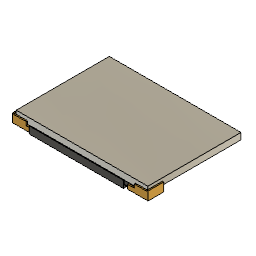
Brackets for Speaker Stand v2 (Autodesk Fusion 360 design; units mm, degrees)
part number: 2026-08-03-13-08-30-619
Autodesk Fusion 360 part; units mm, degrees
sketch "sk REF plate sheet" plane through (0, 0, 0) normal (0, 0, 1) x (1, 0, 0)
  line L0 (-111.75, -122.5) -> (111.75, -122.5)
  line L1 (111.75, -122.5) -> (111.75, 122.5)
  line L2 (111.75, 122.5) -> (-111.75, 122.5)
  line L3 (-111.75, 122.5) -> (-111.75, -122.5)
  dimension "d100" = 111.75
  dimension "d101" = 122.5
  dimension "d102" = 111.75
  dimension "d103" = 122.5
  measures "d100" horizontal distance of origin L0.start
  measures "d101" vertical distance of origin L0.start
  measures "d102" horizontal distance of origin L1.end
  measures "d103" vertical distance of origin L1.end
extrude "REF plate sheet" add sketch "sk REF plate sheet" along normal blind 1.8 makes body 1
sketch "sk REF plate lip" plane through (0, 0, 0) normal (0, 0, 1) x (1, 0, 0)
  line L0 (-111.75, -122.5) -> (111.75, -122.5)
  line L1 (111.75, -122.5) -> (111.75, -120.7)
  line L2 (111.75, -120.7) -> (-111.75, -120.7)
  line L3 (-111.75, -120.7) -> (-111.75, -122.5)
  dimension "d107" = 111.75
  dimension "d108" = 122.5
  dimension "d109" = 111.75
  dimension "d110" = 120.7
  measures "d107" horizontal distance of origin L0.start
  measures "d108" vertical distance of origin L0.start
  measures "d109" horizontal distance of origin L1.end
  measures "d110" vertical distance of origin L1.end
extrude "REF plate lip" add sketch "sk REF plate lip" along normal blind 16.8 bodies 1
fillet "REF plate rear corners" radius 14 2 edges at (111.75, 122.5, 0.9) (-111.75, 122.5, 0.9) on bodies 1
fillet "REF plate lip bend" radius 6 1 edges at (0, -120.7, 1.8) on bodies 1
sketch "sk REF plate holes" plane through (0, 0, 0) normal (0, 0, 1) x (1, 0, 0)
  circle A0 centre (-95.5, -92.5) radius 3
  circle A1 centre (95.5, -92.5) radius 3
  line L0 (-95.5, -92.5) -> (95.5, -92.5) construction
  circle A2 centre (-95.5, 92.5) radius 3
  line L1 (-95.5, -92.5) -> (-95.5, 92.5) construction
  circle A3 centre (95.5, 92.5) radius 3
  line L2 (-95.5, 92.5) -> (95.5, 92.5) construction
  line L3 (95.5, -92.5) -> (95.5, 92.5) construction
  circle A4 centre (0, 0) radius 5
  dimension "d118" = 3
  dimension "d119" = 95.5
  dimension "d120" = 92.5
  dimension "d121" = 191
  dimension "d122" = 185
  dimension "d123" = 5
  constraint equal A0 A1
  constraint horizontal L0
  constraint equal A0 A2
  constraint vertical L1
  constraint equal A0 A3
  constraint horizontal L2
  constraint vertical L3
  constraint coincident A4.centre origin
  measures "d118" radius of A0
  measures "d119" horizontal distance of A4.centre A0.centre
  measures "d120" vertical distance of A4.centre A0.centre
  measures "d121" horizontal distance of A0.centre A1.centre
  measures "d122" vertical distance of A0.centre A2.centre
  measures "d123" radius of A4
extrude "REF plate holes" cut sketch "sk REF plate holes" along normal blind 16.8 bodies 1
sketch "sk REF soft pad strip" plane through (0, 0, 0) normal (0, 0, 1) x (1, 0, 0)
  line L0 (-91.55, -100) -> (-35.55, -100)
  line L1 (-35.55, -100) -> (-35.55, 100)
  line L2 (-35.55, 100) -> (-91.55, 100)
  line L3 (-91.55, 100) -> (-91.55, -100)
  dimension "d127" = 91.55
  dimension "d128" = 100
  dimension "d129" = 35.55
  dimension "d130" = 100
  measures "d127" horizontal distance of origin L0.start
  measures "d128" vertical distance of origin L0.start
  measures "d129" horizontal distance of origin L1.end
  measures "d130" vertical distance of origin L1.end
extrude "REF soft pad strip" add sketch "sk REF soft pad strip" along normal blind 3 from surface at 1.8 separate body makes body 2
mirror "REF soft pad mirror" about plane through (0, 0, 0) normal (1, 0, 0) of bodies 2 makes body 3
sketch "sk 1 tongue over plate" plane through (0, 0, 0) normal (0, 0, 1) x (1, 0, 0)
  line L0 (-160.8, -113.2) -> (-128, -113.2)
  line L1 (-128, -113.2) -> (-104.2, -100)
  line L2 (-104.2, -100) -> (-86.8, -100)
  line L3 (-86.8, -100) -> (-86.8, -85)
  line L4 (-86.8, -85) -> (-104.2, -85)
  line L5 (-104.2, -85) -> (-128, -76)
  line L6 (-128, -76) -> (-160.8, -76)
  line L7 (-160.8, -76) -> (-160.8, -113.2)
  line L8 (-128, -113.2) -> (-128, -76) construction
  line L9 (-104.2, -100) -> (-104.2, -85) construction
  dimension "d136" = 160.8
  dimension "d137" = 128
  dimension "d138" = 104.2
  dimension "d139" = 86.8
  dimension "d140" = 113.2
  dimension "d141" = 100
  dimension "d142" = 85
  dimension "d143" = 76
  constraint vertical L7
  constraint vertical L8
  constraint vertical L9
  constraint vertical L3
  constraint horizontal L0
  constraint horizontal L2
  constraint horizontal L4
  constraint horizontal L6
  measures "d136" horizontal distance of origin L0.start
  measures "d137" horizontal distance of origin L0.end
  measures "d138" horizontal distance of origin L1.end
  measures "d139" horizontal distance of origin L2.end
  measures "d140" vertical distance of origin L0.start
  measures "d141" vertical distance of origin L1.end
  measures "d142" vertical distance of origin L3.end
  measures "d143" vertical distance of origin L5.end
extrude "1 tongue over plate" add sketch "sk 1 tongue over plate" along normal blind 2.6 from surface at 1.8 separate body makes body 4
sketch "sk 2 rib along front" plane through (0, 0, 0) normal (0, 0, 1) x (1, 0, 0)
  line L0 (-160.8, -113.2) -> (-112.05, -113.2)
  line L1 (-112.05, -113.2) -> (-112.05, -110.2)
  line L2 (-112.05, -110.2) -> (-160.8, -110.2)
  line L3 (-160.8, -110.2) -> (-160.8, -113.2)
  dimension "d147" = 160.8
  dimension "d148" = 113.2
  dimension "d149" = 112.05
  dimension "d150" = 110.2
  measures "d147" horizontal distance of origin L0.start
  measures "d148" vertical distance of origin L0.start
  measures "d149" horizontal distance of origin L1.end
  measures "d150" vertical distance of origin L1.end
extrude "2 rib along front" add sketch "sk 2 rib along front" along normal blind 10.4 from surface at -6 bodies 4
sketch "sk 3 rib along back" plane through (0, 0, 0) normal (0, 0, 1) x (1, 0, 0)
  line L0 (-160.8, -79) -> (-112.05, -79)
  line L1 (-112.05, -79) -> (-112.05, -76)
  line L2 (-112.05, -76) -> (-160.8, -76)
  line L3 (-160.8, -76) -> (-160.8, -79)
  dimension "d154" = 160.8
  dimension "d155" = 79
  dimension "d156" = 112.05
  dimension "d157" = 76
  measures "d154" horizontal distance of origin L0.start
  measures "d155" vertical distance of origin L0.start
  measures "d156" horizontal distance of origin L1.end
  measures "d157" vertical distance of origin L1.end
extrude "3 rib along back" add sketch "sk 3 rib along back" along normal blind 10.4 from surface at -6 bodies 4
sketch "sk 4 rib at plate edge is back of C" plane through (0, 0, 0) normal (0, 0, 1) x (1, 0, 0)
  line L0 (-115.05, -113.2) -> (-112.05, -113.2)
  line L1 (-112.05, -113.2) -> (-112.05, -76)
  line L2 (-112.05, -76) -> (-115.05, -76)
  line L3 (-115.05, -76) -> (-115.05, -113.2)
  dimension "d161" = 115.05
  dimension "d162" = 113.2
  dimension "d163" = 112.05
  dimension "d164" = 76
  measures "d161" horizontal distance of origin L0.start
  measures "d162" vertical distance of origin L0.start
  measures "d163" horizontal distance of origin L1.end
  measures "d164" vertical distance of origin L1.end
extrude "4 rib at plate edge is back of C" add sketch "sk 4 rib at plate edge is back of C" along normal blind 10.4 from surface at -6 bodies 4
sketch "sk 5 flange under plate" plane through (0, 0, 0) normal (0, 0, 1) x (1, 0, 0)
  line L0 (-112.05, -104.5) -> (-86.8, -104.5)
  line L1 (-86.8, -104.5) -> (-86.8, -80.5)
  line L2 (-86.8, -80.5) -> (-112.05, -80.5)
  line L3 (-112.05, -80.5) -> (-112.05, -104.5)
  dimension "d168" = 112.05
  dimension "d169" = 104.5
  dimension "d170" = 86.8
  dimension "d171" = 80.5
  measures "d168" horizontal distance of origin L0.start
  measures "d169" vertical distance of origin L0.start
  measures "d170" horizontal distance of origin L1.end
  measures "d171" vertical distance of origin L1.end
extrude "5 flange under plate" add sketch "sk 5 flange under plate" along normal blind 5.6 from surface at -6 bodies 4
sketch "sk 6 side wall is left-right stop" plane through (0, 0, 0) normal (0, 0, 1) x (1, 0, 0)
  line L0 (-160.8, -113.2) -> (-157.8, -113.2)
  line L1 (-157.8, -113.2) -> (-157.8, -76)
  line L2 (-157.8, -76) -> (-160.8, -76)
  line L3 (-160.8, -76) -> (-160.8, -113.2)
  dimension "d175" = 160.8
  dimension "d176" = 113.2
  dimension "d177" = 157.8
  dimension "d178" = 76
  measures "d175" horizontal distance of origin L0.start
  measures "d176" vertical distance of origin L0.start
  measures "d177" horizontal distance of origin L1.end
  measures "d178" vertical distance of origin L1.end
extrude "6 side wall is left-right stop" add sketch "sk 6 side wall is left-right stop" along normal blind 20.8 from surface at -6 bodies 4
sketch "sk 7 front wall is fore-aft stop" plane through (0, 0, 0) normal (0, 0, 1) x (1, 0, 0)
  line L0 (-160.8, -113.2) -> (-128, -113.2)
  line L1 (-128, -113.2) -> (-128, -110.2)
  line L2 (-128, -110.2) -> (-160.8, -110.2)
  line L3 (-160.8, -110.2) -> (-160.8, -113.2)
  dimension "d182" = 160.8
  dimension "d183" = 113.2
  dimension "d184" = 128
  dimension "d185" = 110.2
  measures "d182" horizontal distance of origin L0.start
  measures "d183" vertical distance of origin L0.start
  measures "d184" horizontal distance of origin L1.end
  measures "d185" vertical distance of origin L1.end
extrude "7 front wall is fore-aft stop" add sketch "sk 7 front wall is fore-aft stop" along normal blind 18.8 from surface at -6 bodies 4
sketch "sk 8 M3 screw slot" plane through (0, 0, 0) normal (0, 0, 1) x (1, 0, 0)
  line L0 (-100.75, -94.25) -> (-90.25, -94.25)
  line L1 (-90.25, -94.25) -> (-90.25, -90.75)
  line L2 (-90.25, -90.75) -> (-100.75, -90.75)
  line L3 (-100.75, -90.75) -> (-100.75, -94.25)
  dimension "d189" = 100.75
  dimension "d190" = 94.25
  dimension "d191" = 90.25
  dimension "d192" = 90.75
  measures "d189" horizontal distance of origin L0.start
  measures "d190" vertical distance of origin L0.start
  measures "d191" horizontal distance of origin L1.end
  measures "d192" vertical distance of origin L1.end
extrude "8 M3 screw slot" cut sketch "sk 8 M3 screw slot" along normal blind 10.4 from surface at -6 bodies 4
sketch "sk 9 M3 head counterbore" plane through (0, 0, 0) normal (0, 0, 1) x (1, 0, 0)
  line L0 (-102.2, -95.7) -> (-88.8, -95.7)
  line L1 (-88.8, -95.7) -> (-88.8, -89.3)
  line L2 (-88.8, -89.3) -> (-102.2, -89.3)
  line L3 (-102.2, -89.3) -> (-102.2, -95.7)
  dimension "d196" = 102.2
  dimension "d197" = 95.7
  dimension "d198" = 88.8
  dimension "d199" = 89.3
  measures "d196" horizontal distance of origin L0.start
  measures "d197" vertical distance of origin L0.start
  measures "d198" horizontal distance of origin L1.end
  measures "d199" vertical distance of origin L1.end
extrude "9 M3 head counterbore" cut sketch "sk 9 M3 head counterbore" along normal blind 1.8 from surface at 2.6 bodies 4
sketch "sk 10 M3 nut channel" plane through (0, 0, 0) normal (0, 0, 1) x (1, 0, 0)
  line L0 (-102.05, -95.4) -> (-88.95, -95.4)
  line L1 (-88.95, -95.4) -> (-88.95, -89.6)
  line L2 (-88.95, -89.6) -> (-102.05, -89.6)
  line L3 (-102.05, -89.6) -> (-102.05, -95.4)
  dimension "d203" = 102.05
  dimension "d204" = 95.4
  dimension "d205" = 88.95
  dimension "d206" = 89.6
  measures "d203" horizontal distance of origin L0.start
  measures "d204" vertical distance of origin L0.start
  measures "d205" horizontal distance of origin L1.end
  measures "d206" vertical distance of origin L1.end
extrude "10 M3 nut channel" cut sketch "sk 10 M3 nut channel" along normal blind 2.6 from surface at -6 bodies 4
mirror "11 mirror to right side" about plane through (0, 0, 0) normal (1, 0, 0) of bodies 4 makes body 5
sketch "sk REF MacBook Pro 14 envelope" plane through (0, 0, 0) normal (0, 0, 1) x (1, 0, 0)
  line L0 (-156.3, -109.2) -> (156.3, -109.2)
  line L1 (156.3, -109.2) -> (156.3, 112)
  line L2 (156.3, 112) -> (-156.3, 112)
  line L3 (-156.3, 112) -> (-156.3, -109.2)
  dimension "d212" = 156.3
  dimension "d213" = 109.2
  dimension "d214" = 156.3
  dimension "d215" = 112
  measures "d212" horizontal distance of origin L0.start
  measures "d213" vertical distance of origin L0.start
  measures "d214" horizontal distance of origin L1.end
  measures "d215" vertical distance of origin L1.end
extrude "REF MacBook Pro 14 envelope" add sketch "sk REF MacBook Pro 14 envelope" along normal blind 15.5 from surface at 4.8 separate body makes body 6
equation "plate_width = 223.5 mm" comment "[EST] left-right; the lip runs along this edge"
equation "plate_depth = 245 mm" comment "[EST] front-back"
equation "plate_thickness = 1.8 mm" comment "[EST] sheet gauge"
equation "plate_rear_corner_radius = 14 mm" comment "[EST] rear corners only; lip corners are square"
equation "lip_height_above_plate = 15 mm" comment "[EST] flat height above the plate top face"
equation "lip_bend_radius = 6 mm" comment "MEASURED inside radius, vertical section"
equation "hole_diameter = 6 mm" comment "[EST]"
equation "hole_spacing_left_right = 191 mm" comment "[EST] centre-to-centre across the plate"
equation "hole_spacing_front_back = 185 mm" comment "[EST] centre-to-centre along the plate"
equation "centre_boss_diameter = 10 mm" comment "nominal, the M8 tilt-screw slot"
equation "softpad_thickness = 3 mm" comment "[EST] governs the whole bracket section"
equation "softpad_outer_edge_inset = 20.2 mm" comment "[EST] strip outer edge, in from the plate side edge"
equation "softpad_strip_width = 56 mm" comment "[EST] X width of each strip"
equation "softpad_strip_length = 200 mm" comment "[EST] Y length of each strip"
equation "laptop_width = 312.6 mm" comment "MEASURED Apple spec, 14in MacBook Pro"
equation "laptop_depth = 221.2 mm" comment "MEASURED"
equation "laptop_height = 15.5 mm" comment "MEASURED"
equation "screw_clearance_radius = 1.75 mm" comment "M3 shank clearance"
equation "screw_head_radius = 3.2 mm" comment "M3 button head is 5.7 dia"
equation "screw_head_height = 1.8 mm" comment "counterbore depth"
equation "screw_slot_travel = 3.5 mm" comment "+/- along X; absorbs hole-spacing error"
equation "nut_across_flats = 5.5 mm" comment "M3"
equation "nut_thickness = 2.4 mm"
equation "nut_pocket_clearance = 0.3 mm" comment "so the nut drops in but cannot rotate"
equation "nut_pocket_extra_depth = 0.2 mm"
equation "laptop_side_clearance = 1.5 mm" comment "per side, laptop edge to wall"
equation "laptop_front_clearance = 1 mm" comment "laptop nose to front wall"
equation "tongue_clearance = 0.4 mm" comment "tongue sits this far below the laptop"
equation "wall_thickness = 3 mm"
equation "side_wall_height = 10 mm" comment "above the laptop underside"
equation "front_wall_height = 8 mm" comment "lower: it is nearer the lid edge"
equation "front_wall_length = 32.8 mm" comment "how far along X the front wall runs"
equation "lip_bend_clearance = 1.5 mm" comment "keep the front wall off the bend radius"
equation "plate_edge_clearance = 0.3 mm" comment "slip fit against the plate outer edge"
equation "rib_depth_below_plate = 6 mm" comment "how far the whole underside hangs down"
equation "rib_thickness = 3 mm"
equation "boss_wall = 2 mm" comment "material around the counterbore"
equation "bracket_depth_behind_hole = 16.5 mm" comment "back edge of the corner block"
equation "boss_half_depth = 7.5 mm" comment "Y half-height of the bolt boss"
equation "plate_grip_clearance = 0.4 mm" comment "gap under the plate before the flange bears"
equation "flange_width = 24 mm" comment "lower flange, the other half of the C"
equation "plate_half_width = plate_width / 2"
equation "plate_half_depth = plate_depth / 2"
equation "plate_edge_x = plate_half_width + plate_edge_clearance" comment "bracket sits just outside this"
equation "lip_top_z = plate_thickness + lip_height_above_plate"
equation "lip_inner_y = plate_half_depth - plate_thickness" comment "lip inner face"
equation "plate_flat_front_y = lip_inner_y - lip_bend_radius" comment "plate top is flat only behind this"
equation "hole_x = hole_spacing_left_right / 2"
equation "hole_front_y = hole_spacing_front_back / 2" comment "the lip-side holes -- the ones used"
equation "hole_radius = hole_diameter / 2"
equation "centre_boss_radius = centre_boss_diameter / 2"
equation "softpad_outer_x = plate_half_width - softpad_outer_edge_inset"
equation "softpad_inner_x = softpad_outer_x - softpad_strip_width"
equation "softpad_half_length = softpad_strip_length / 2"
equation "tongue_thickness = softpad_thickness - tongue_clearance" comment "only material under the laptop"
equation "tongue_top_z = plate_thickness + tongue_thickness"
equation "laptop_underside_z = plate_thickness + softpad_thickness" comment "laptop rests on the stock pads"
equation "flange_top_z = plate_grip_clearance" comment "below Z0"
equation "flange_bottom_z = rib_depth_below_plate" comment "below Z0"
equation "flange_thickness = rib_depth_below_plate - plate_grip_clearance"
equation "throat_height = plate_thickness + plate_grip_clearance" comment "the C throat"
equation "counterbore_floor = tongue_thickness - screw_head_height" comment "CHECK keep above 0.8"
equation "nut_pocket_depth = nut_thickness + nut_pocket_extra_depth"
equation "nut_pocket_floor = flange_thickness - nut_pocket_depth" comment "CHECK keep above 1.5"
equation "front_wall_outer_y = plate_flat_front_y - lip_bend_clearance"
equation "front_wall_inner_y = front_wall_outer_y - wall_thickness"
equation "laptop_front_y = front_wall_inner_y - laptop_front_clearance"
equation "laptop_rear_y = laptop_depth - laptop_front_y" comment "signed +Y"
equation "laptop_half_width = laptop_width / 2"
equation "lip_to_laptop_gap = lip_inner_y - laptop_front_y" comment "CHECK keep above 6"
equation "rear_margin = plate_half_depth - laptop_rear_y" comment "CHECK keep above 5"
equation "side_wall_inner_x = laptop_half_width + laptop_side_clearance"
equation "side_wall_outer_x = side_wall_inner_x + wall_thickness"
equation "cantilever = side_wall_outer_x - plate_half_width" comment "unsupported reach"
equation "bracket_back_y = hole_front_y - bracket_depth_behind_hole"
equation "rib_back_outer_y = bracket_back_y + rib_thickness"
equation "rib_edge_outer_x = plate_edge_x + rib_thickness"
equation "front_wall_end_x = side_wall_outer_x - front_wall_length"
equation "boss_outer_x = hole_x + screw_slot_travel + screw_head_radius + boss_wall"
equation "boss_inner_x = hole_x - screw_slot_travel - screw_head_radius - boss_wall"
equation "boss_front_y = hole_front_y + boss_half_depth"
equation "boss_back_y = hole_front_y - boss_half_depth"
equation "boss_pad_overlap = softpad_outer_x - boss_inner_x" comment "CHECK above 0 = boss sits on the pad"
equation "flange_front_y = hole_front_y + flange_width / 2"
equation "flange_back_y = hole_front_y - flange_width / 2"
equation "slot_outer_x = hole_x + screw_slot_travel + screw_clearance_radius"
equation "slot_inner_x = hole_x - screw_slot_travel - screw_clearance_radius"
equation "slot_front_y = hole_front_y + screw_clearance_radius"
equation "slot_back_y = hole_front_y - screw_clearance_radius"
equation "cbore_outer_x = hole_x + screw_slot_travel + screw_head_radius"
equation "cbore_inner_x = hole_x - screw_slot_travel - screw_head_radius"
equation "cbore_front_y = hole_front_y + screw_head_radius"
equation "cbore_back_y = hole_front_y - screw_head_radius"
equation "nut_pocket_x_half = screw_slot_travel + nut_across_flats / 2 + nut_pocket_clearance"
equation "nut_pocket_y_half = ( nut_across_flats + nut_pocket_clearance ) / 2"
equation "nut_pocket_outer_x = hole_x + nut_pocket_x_half"
equation "nut_pocket_inner_x = hole_x - nut_pocket_x_half"
equation "nut_pocket_front_y = hole_front_y + nut_pocket_y_half"
equation "nut_pocket_back_y = hole_front_y - nut_pocket_y_half"
equation "d100 = plate_half_width"
equation "d101 = plate_half_depth"
equation "d102 = plate_half_width"
equation "d103 = plate_half_depth"
equation "d105 = plate_thickness"
equation "d107 = plate_half_width"
equation "d108 = plate_half_depth"
equation "d109 = plate_half_width"
equation "d110 = lip_inner_y"
equation "d112 = lip_top_z"
equation "d115 = plate_rear_corner_radius"
equation "d117 = lip_bend_radius"
equation "d118 = hole_radius"
equation "d119 = hole_x"
equation "d120 = hole_front_y"
equation "d121 = hole_spacing_left_right"
equation "d122 = hole_spacing_front_back"
equation "d123 = centre_boss_radius"
equation "d125 = lip_top_z"
equation "d127 = softpad_outer_x"
equation "d128 = softpad_half_length"
equation "d129 = softpad_inner_x"
equation "d130 = softpad_half_length"
equation "d131 = plate_thickness"
equation "d132 = softpad_thickness"
equation "d136 = side_wall_outer_x"
equation "d137 = front_wall_end_x"
equation "d138 = boss_outer_x"
equation "d139 = boss_inner_x"
equation "d140 = front_wall_outer_y"
equation "d141 = boss_front_y"
equation "d142 = boss_back_y"
equation "d143 = bracket_back_y"
equation "d144 = plate_thickness"
equation "d145 = tongue_thickness"
equation "d147 = side_wall_outer_x"
equation "d148 = front_wall_outer_y"
equation "d149 = plate_edge_x"
equation "d150 = front_wall_inner_y"
equation "d151 = -rib_depth_below_plate"
equation "d152 = tongue_top_z + rib_depth_below_plate"
equation "d154 = side_wall_outer_x"
equation "d155 = rib_back_outer_y"
equation "d156 = plate_edge_x"
equation "d157 = bracket_back_y"
equation "d158 = -rib_depth_below_plate"
equation "d159 = tongue_top_z + rib_depth_below_plate"
equation "d161 = rib_edge_outer_x"
equation "d162 = front_wall_outer_y"
equation "d163 = plate_edge_x"
equation "d164 = bracket_back_y"
equation "d165 = -rib_depth_below_plate"
equation "d166 = tongue_top_z + rib_depth_below_plate"
equation "d168 = plate_edge_x"
equation "d169 = flange_front_y"
equation "d170 = boss_inner_x"
equation "d171 = flange_back_y"
equation "d172 = -flange_bottom_z"
equation "d173 = flange_thickness"
equation "d175 = side_wall_outer_x"
equation "d176 = front_wall_outer_y"
equation "d177 = side_wall_inner_x"
equation "d178 = bracket_back_y"
equation "d179 = -rib_depth_below_plate"
equation "d180 = rib_depth_below_plate + laptop_underside_z + side_wall_height"
equation "d182 = side_wall_outer_x"
equation "d183 = front_wall_outer_y"
equation "d184 = front_wall_end_x"
equation "d185 = front_wall_inner_y"
equation "d186 = -rib_depth_below_plate"
equation "d187 = rib_depth_below_plate + laptop_underside_z + front_wall_height"
equation "d189 = slot_outer_x"
equation "d190 = slot_front_y"
equation "d191 = slot_inner_x"
equation "d192 = slot_back_y"
equation "d193 = -flange_bottom_z"
equation "d194 = flange_bottom_z + tongue_top_z"
equation "d196 = cbore_outer_x"
equation "d197 = cbore_front_y"
equation "d198 = cbore_inner_x"
equation "d199 = cbore_back_y"
equation "d200 = tongue_top_z - screw_head_height"
equation "d201 = screw_head_height"
equation "d203 = nut_pocket_outer_x"
equation "d204 = nut_pocket_front_y"
equation "d205 = nut_pocket_inner_x"
equation "d206 = nut_pocket_back_y"
equation "d207 = -flange_bottom_z"
equation "d208 = nut_pocket_depth"
equation "d212 = laptop_half_width"
equation "d213 = laptop_front_y"
equation "d214 = laptop_half_width"
equation "d215 = laptop_rear_y"
equation "d216 = laptop_underside_z"
equation "d217 = laptop_height"
named bodies: "plate", "REF soft pad", "REF soft pad (1)", "corner bracket", "corner bracket (1)", "REF MacBook Pro 14"
